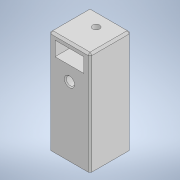
# Autodesk Inventor part: Idle Bearing Mount
Saved by Autodesk Inventor 2022 (Build 260153000, 153)
## iProperties
Created: 2022-04-23
Part Number: Idle Bearing Mount
Material: Generic
Document SubType Name: Modeling
Designer: Nick
Density: 1 g/cm^3
Appearance: Default
Author: Nick
Autodesk Inventor part; units mm, degrees
ref_plane "YZ Plane" through (0, 0, 0) normal (1, 0, 0) x (0, 1, 0)
ref_plane "XZ Plane" through (0, 0, 0) normal (0, 1, 0) x (-1, 0, 0)
ref_plane "XY Plane" through (0, 0, 0) normal (0, 0, 1) x (1, 0, 0)
sketch "Sketch1" plane through (0, 0, 0) normal (0, 0, 1) x (1, 0, 0)
  line L0 (0, 50) -> (20, 50)
  line L1 (20, 50) -> (20, 0)
  line L2 (20, 0) -> (0, 0)
  line L3 (0, 0) -> (0, 50)
  line L4 (3, 47.5) -> (17, 47.5)
  line L5 (17, 47.5) -> (17, 40.5)
  line L6 (17, 40.5) -> (3, 40.5)
  line L7 (3, 40.5) -> (3, 47.5)
  point P0 (10, 47.5)
  point P1 (10, 50)
  dimension "d1" = 20
  dimension "d2" = 14
  dimension "d3" = 7
  dimension "d4" = 2.5
  dimension "d66" = 40.5
  constraints: 16 end point, 4 parallel, 2 horizontal, 2 midpoint, 2 perpendicular, 1 coincident, 1 vertical alignment
  measures "d1" distance of L1.end L2.end
  measures "d2" distance of L4.start L4.end
  measures "d3" distance of L4.end L5.end
  measures "d4" distance between parallel lines of L4 L0
  measures "d66" distance between parallel lines of L2 L6
extrude "Extrusion1" add sketch "Sketch1" along normal blind 20
sketch "Sketch2" plane through (0, 0, 0) normal (0, -1, 0) x (1, 0, 0)
  line L0 (0, 0) -> (20, 0) projected
  line L1 (20, 0) -> (20, 20) projected
  line L2 (0, 0) -> (0, 20) projected
  line L3 (0, 20) -> (20, 20) projected
  point P0 (10, 4)
  point P1 (16, 16)
  point P2 (4, 16)
  point P3 (10, 0)
  dimension "d9" = 4
  dimension "d12" = 4
  dimension "d13" = 4
  dimension "d14" = 4
  constraints: 1 horizontal alignment, 1 midpoint, 1 vertical alignment
  measures "d9" distance from line of L0 point (10, 4)
  measures "d12" distance from line of L1 point (16, 16)
  measures "d13" distance from line of L3 point (16, 16)
  measures "d14" distance from line of L2 point (4, 16)
hole "Hole1" at (10, 0, 4) at (16, 0, 16) at (4, 0, 16) direction (0, 1, 0) diameter 4 depth 7
sketch "Sketch3" plane through (0, 0, 20) normal (0, 0, 1) x (1, 0, 0)
  line L0 (17, 40.5) -> (3, 40.5) projected
  point P0 (0, 0)
  point P1 (10, 33.5)
  point P2 (10, 40.5)
  dimension "d22" = 7
  constraints: 1 midpoint, 1 vertical alignment
  measures "d22" distance from line of L0 point (10, 33.5)
hole "Hole2" at (10, 33.5, 20) direction (0, 0, -1) diameter 4 depth 6
chamfer "Chamfer1" distance 0.5 angle 45 1 edges at (10, 35.5, 20)
sketch "Sketch4" plane through (0, 50, 0) normal (0, 1, 0) x (1, 0, 0)
  line L0 (8, -14) -> (12, -14) projected
  line L1 (12, -19.5) -> (8, -19.5) projected
  line L2 (20, 0) -> (0, 0) projected
  point P0 (10, -7)
  point P1 (10, 0)
  dimension "d33" = 7
  dimension "d34" = 7
  constraints: 1 midpoint, 1 vertical alignment
  measures "d33" distance from line of L0 point (10, -7)
  measures "d34" distance from line of L2 point (10, -7)
hole "Hole3" at (10, 50, 7) direction (0, -1, 0) diameter 3.4 depth 20 clearance for "Socket Head Cap Screw" size "M3" standard "Ansi Metric M Profile"
sketch "Sketch5" plane through (3, 40.5, 0) normal (0, 1, 0) x (1, 0, 0)
  circle A0 centre (7, -7) radius 1.7 projected
  circle A1 centre (7, -7) radius 2.5
  point P0 (-3, 0)
  dimension "d42" = 5
  constraints: 1 centre point, 1 coincident
  measures "d42" diameter of A1
extrude "Extrusion2" add sketch "Sketch5" along normal blind 0.95
chamfer "Chamfer2" distance 0.95 angle 45 1 edges at (7.5, 40.5, 7)
sketch "Sketch6" plane through (3, 47.5, 0) normal (0, -1, 0) x (1, 0, 0)
  circle A0 centre (7, 7) radius 1.7 projected
  circle A1 centre (7, 7) radius 2.5
  point P0 (-3, 0)
  dimension "d48" = 5
  constraints: 1 centre point, 1 coincident
  measures "d48" diameter of A1
extrude "Extrusion3" add sketch "Sketch6" along normal blind 0.95
chamfer "Chamfer3" distance 0.95 angle 45 1 edges at (7.5, 47.5, 7)
sketch "Sketch7" plane through (0, 0, 0) normal (0, -1, 0) x (1, 0, 0)
  circle A0 centre (16, 16) radius 2 projected
  circle A1 centre (10, 4) radius 2 projected
  circle A2 centre (4, 16) radius 2 projected
  line L0 (0, 0) -> (20, 0) projected
  line L1 (20, 0) -> (20, 20) projected
  line L2 (0, 20) -> (20, 20) projected
  line L3 (0, 0) -> (0, 20) projected
  line L4 (15, 17.7321) -> (16, 18.3094)
  line L5 (16, 18.3094) -> (17, 17.7321)
  line L6 (3, 17.7321) -> (4, 18.3094)
  line L7 (4, 18.3094) -> (5, 17.7321)
  line L8 (9, 5.7321) -> (10, 6.3094)
  line L9 (10, 6.3094) -> (11, 5.7321)
  circle A3 centre (10, 4) radius 2 projected
  circle A4 centre (10, 4) radius 2 construction
  line L10 (10, 6.3094) -> (10, 4) construction
  circle A5 centre (16, 16) radius 2 construction
  line L11 (16, 18.3094) -> (16, 16) construction
  line L12 (4, 18.3094) -> (4, 16) construction
  dimension "d54" = 120
  dimension "d55" = 120
  dimension "d56" = 120
  constraints: 18 end point, 4 point on circle, 4 tangent, 3 vertical, 6 other
  measures "d54" angle of L8 L9
  measures "d55" angle of L5 L4
  measures "d56" angle of L7 L6
extrude "Extrusion4" cut sketch "Sketch7" against normal up to surface (7 mm away) contours A0 L4 L5 | A1 L8 L9 | A2 L6 L7
ref_plane "Work Plane2" through (3, 36.5, 0) normal (0, 1, 0) x (1, 0, 0)
sketch "Sketch8" plane through (3, 36.5, 0) normal (0, 1, 0) x (1, 0, 0)
  circle A0 centre (7, -7) radius 1.7 projected
  circle A1 centre (7, -7) radius 1.7 projected
  line L0 (4.25, -5.4123) -> (7, -3.8246)
  line L1 (7, -3.8246) -> (9.75, -5.4123)
  line L2 (9.75, -5.4123) -> (9.75, -8.5877)
  line L3 (9.75, -8.5877) -> (7, -10.1754)
  line L4 (7, -10.1754) -> (4.25, -8.5877)
  line L5 (4.25, -8.5877) -> (4.25, -5.4123)
  line L6 (9.75, -5.4123) -> (9.75, 0.1245)
  line L7 (4.25, -5.4123) -> (4.25, 0)
  line L8 (0, 0) -> (14, 0) projected
  point P0 (-3, 0)
  point P1 (7, -7)
  point P2 (9.75, 0)
  dimension "d60" = 5.5
  constraints: 16 end point, 2 vertical, 1 coincident, 1 point on line, 15 other
  measures "d60" distance between parallel lines of L5 L2
extrude "Extrusion5" cut sketch "Sketch8" against normal blind 2.5
chamfer "Chamfer4" distance 0.95 angle 45 8 edges at (0, 25, 20) (20, 25, 20) (10, 50, 20) (10, 50, 0) (0, 25, 0) (20, 25, 0) (20, 50, 10) (0, 50, 10)
equation "\"d9\" = d12"
equation "\"d13\" = d12"
equation "\"d14\" = d12"
equation "\"d33\" = d34"
equation "\"MotorHeight\" = MotorHeightBase"
equation "\"MotorHeightBase\" = 32"
body "Solid1"
